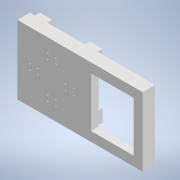
# Autodesk Inventor part: Upper_Half
Saved by Autodesk Inventor 2022 (Build 260153000, 153)
## iProperties
Created: 2023-09-02
Part Number: Upper_Half
Material: Generic
Document SubType Name: Modeling
Designer: Petr Černý
Density: 1 g/cm^3
Appearance: Default
Author: Petr Černý
Autodesk Inventor part; units mm, degrees
ref_plane "YZ Plane" through (0, 0, 0) normal (1, 0, 0) x (0, 1, 0)
ref_plane "XZ Plane" through (0, 0, 0) normal (0, 1, 0) x (-1, 0, 0)
ref_plane "XY Plane" through (0, 0, 0) normal (0, 0, 1) x (1, 0, 0)
sketch "Sketch1" plane through (0, 0, 0) normal (0, 0, 1) x (1, 0, 0)
  line L0 (99.9399, 34.6241) -> (-14.0601, 34.6241)
  line L1 (-14.0601, 34.6241) -> (-14.0601, -20.3759)
  line L2 (-14.0601, -20.3759) -> (99.9399, -20.3759)
  line L3 (99.9399, -20.3759) -> (99.9399, 34.6241)
  point P0 (0, 0)
  dimension "d0" = 114
  dimension "d1" = 55
  constraints: 8 end point, 2 parallel, 1 horizontal, 1 perpendicular
  measures "d0" distance of L1.end L2.end
  measures "d1" distance of L0.end L1.end
extrude "Extrusion1" add sketch "Sketch1" along normal blind 6
shell "Shell1" thickness 2 removed faces 1 at (23.9399, -2.0426, 0)
sketch "Sketch2" plane through (97.9399, 32.6241, 4) normal (0, 0, -1) x (-1, 0, 0)
  line L0 (110, 0) -> (110, -51) projected
  line L1 (0, 0) -> (110, 0) projected
  line L2 (110, 0) -> (110, -51) projected
  line L3 (110, -51) -> (0, -51) projected
  line L4 (0, -51) -> (0, 0) projected
  line L5 (112, 2) -> (112, -53) projected
  line L6 (-2, 2) -> (112, 2) projected
  line L7 (-2, -53) -> (-2, 2) projected
  line L8 (112, -53) -> (-2, -53) projected
  line L9 (110, 0) -> (110, -51) projected
  line L10 (110, 0) -> (100, 0)
  line L11 (100, 0) -> (100, -10)
  line L12 (100, -10) -> (110, -10)
  line L13 (110, -10) -> (110, 0)
  line L14 (110, -51) -> (0, -51) projected
  line L15 (110, -51) -> (100, -51)
  line L16 (100, -51) -> (100, -41)
  line L17 (100, -41) -> (110, -41)
  line L18 (110, -41) -> (110, -51)
  line L19 (0, 0) -> (110, 0) projected
  line L20 (70, 0) -> (60, 0)
  line L21 (60, 0) -> (60, -10)
  line L22 (60, -10) -> (70, -10)
  line L23 (70, -10) -> (70, 0)
  line L24 (70, -51) -> (60, -51)
  line L25 (60, -51) -> (60, -41)
  line L26 (60, -41) -> (70, -41)
  line L27 (70, -41) -> (70, -51)
  point P0 (97.9399, -32.6241)
  point P1 (105, -4.45)
  point P2 (105, -46.55)
  point P3 (65, -4.45)
  point P4 (65, -46.55)
  point P5 (60, 0)
  point P6 (100, 0)
  dimension "d5" = 10
  dimension "d6" = 10
  dimension "d7" = 10
  dimension "d8" = 10
  dimension "d9" = 10
  dimension "d10" = 10
  dimension "d11" = 10
  dimension "d12" = 10
  dimension "d13" = 30
  dimension "d14" = 4.45
  dimension "d15" = 4.45
  dimension "d16" = 42.1
  dimension "d17" = 5
  dimension "d18" = 5
  dimension "d19" = 40
  dimension "d20" = 40
  constraints: 32 end point, 8 parallel, 4 horizontal, 4 perpendicular, 3 point on line
  measures "d5" distance of L12.end L11.end
  measures "d6" distance of L11.end L10.end
  measures "d7" distance of L16.end L17.end
  measures "d8" distance of L15.end L16.end
  measures "d9" distance of L22.end L21.end
  measures "d10" distance of L21.end L20.end
  measures "d11" distance of L25.end L26.end
  measures "d12" distance of L24.end L25.end
  measures "d13" distance between parallel lines of L11 L23
  measures "d14" distance from line of L1 point (105, -4.45)
  measures "d15" distance from line of L3 point (105, -46.55)
  measures "d16" distance of point (105, -46.55) point (105, -4.45)
  measures "d17" distance from line of L0 point (105, -4.45)
  measures "d18" distance from line of L0 point (105, -46.55)
  measures "d19" distance of point (65, -4.45) point (105, -4.45)
  measures "d20" distance of point (65, -46.55) point (105, -46.55)
extrude "Extrusion2" add sketch "Sketch2" along normal blind 14 contours L0 L12 L11 L1 | L0 L3 L16 L17 | L23 L22 L21 L1 | L3 L25 L26 L27
sketch "Sketch3" plane through (0, 0, 0) normal (0, 0, -1) x (-1, 0, 0)
  line L0 (-27.9399, -18.3759) -> (-37.9399, -18.3759) projected
  line L1 (12.0601, -8.3759) -> (12.0601, -18.3759) projected
  line L2 (2.0601, -18.3759) -> (2.0601, -8.3759) projected
  line L3 (-27.9399, -8.3759) -> (-27.9399, -18.3759) projected
  point P0 (0, 0)
  point P1 (7.0601, 28.1741)
  point P2 (7.0601, -13.9259)
  point P3 (-32.9399, -13.9259)
  point P4 (-32.9399, 28.1741)
  point P5 (7.0601, 28.1741)
  point P6 (7.0601, -13.9259)
  point P7 (-32.9399, -13.9259)
  point P8 (-32.9399, 28.1741)
  dimension "d66" = 42.1
  dimension "d67" = 4.45
  dimension "d68" = 40
  dimension "d69" = 5
  dimension "d70" = 30
  constraints: 4 coincident
  measures "d66" distance of point (-32.94, -13.926) point (-32.94, 28.174)
  measures "d67" distance from line of L0 point (-32.94, -13.926)
  measures "d68" distance of point (7.06, -13.926) point (-32.94, -13.926)
  measures "d69" distance from line of L1 point (7.06, -13.926)
  measures "d70" distance between parallel lines of L2 L3
hole "Hole1" at (-7.0601, 28.1741, 0) at (-7.0601, -13.9259, 0) at (32.9399, -13.9259, 0) at (32.9399, 28.1741, 0) direction (0, 0, 1) diameter 2.459 depth 5 tip angle 118 thread size "M3x0.5" class "6H" standard "ISO Metric profile"
sketch "Sketch4" plane through (0, 0, 6) normal (0, 0, 1) x (1, 0, 0)
  line L0 (-14.0601, 34.6241) -> (-14.0601, -20.3759) projected
  line L1 (99.9399, 34.6241) -> (-14.0601, 34.6241) projected
  line L2 (-14.0601, -20.3759) -> (99.9399, -20.3759) projected
  point P0 (0, 0)
  point P1 (-4.0601, 9.3741)
  point P2 (-4.0601, 4.8741)
  point P3 (2.4399, 4.8741)
  point P4 (2.4399, 9.3741)
  point P5 (10.1899, -5.1259)
  point P6 (10.1899, -9.6259)
  point P7 (16.6899, -9.6259)
  point P8 (16.6899, -5.1259)
  point P9 (16.6899, 23.8741)
  point P10 (16.6899, 19.3741)
  point P11 (10.1899, 19.3741)
  point P12 (10.1899, 23.8741)
  point P13 (30.9399, 9.3741)
  point P14 (24.4399, 9.3741)
  point P15 (24.4399, 4.8741)
  point P16 (30.9399, 4.8741)
  dimension "d30" = 4.5
  dimension "d31" = 6.5
  dimension "d32" = 6.5
  dimension "d33" = 10
  dimension "d34" = 25.25
  dimension "d35" = 4.5
  dimension "d36" = 6.5
  dimension "d37" = 6.5
  dimension "d38" = 4.5
  dimension "d39" = 6.5
  dimension "d40" = 6.5
  dimension "d41" = 4.5
  dimension "d42" = 6.5
  dimension "d43" = 6.5
  dimension "d44" = 22
  dimension "d45" = 0
  dimension "d46" = 7.75
  dimension "d47" = 7.75
  dimension "d48" = 10
  dimension "d49" = 10
  measures "d30" distance of point (-4.06, 4.874) point (-4.06, 9.374)
  measures "d31" distance of point (2.44, 9.374) point (-4.06, 9.374)
  measures "d32" distance of point (2.44, 4.874) point (-4.06, 4.874)
  measures "d33" distance from line of L0 point (-4.06, 4.874)
  measures "d34" distance from line of L2 point (-4.06, 4.874)
  measures "d35" distance of point (10.19, -9.626) point (10.19, -5.126)
  measures "d36" distance of point (16.69, -5.126) point (10.19, -5.126)
  measures "d37" distance of point (16.69, -9.626) point (10.19, -9.626)
  measures "d38" distance of point (10.19, 19.374) point (10.19, 23.874)
  measures "d39" distance of point (16.69, 23.874) point (10.19, 23.874)
  measures "d40" distance of point (16.69, 19.374) point (10.19, 19.374)
  measures "d41" distance of point (24.44, 4.874) point (24.44, 9.374)
  measures "d42" distance of point (30.94, 9.374) point (24.44, 9.374)
  measures "d43" distance of point (30.94, 4.874) point (24.44, 4.874)
  measures "d44" distance of point (24.44, 4.874) point (2.44, 4.874)
  measures "d45" vertical distance of point (24.44, 4.874) point (2.44, 4.874)
  measures "d46" horizontal distance of point (10.19, -9.626) point (2.44, 4.874)
  measures "d47" horizontal distance of point (10.19, 19.374) point (2.44, 9.374)
  measures "d48" vertical distance of point (2.44, 9.374) point (10.19, 19.374)
  measures "d49" vertical distance of point (10.19, -5.126) point (2.44, 4.874)
hole "Hole2" at (-4.0601, 9.3741, 6) at (-4.0601, 4.8741, 6) at (2.4399, 4.8741, 6) at (2.4399, 9.3741, 6) at (16.6899, -5.1259, 6) at (16.6899, -9.6259, 6) at (10.1899, -9.6259, 6) at (10.1899, -5.1259, 6) at (16.6899, 23.8741, 6) at (10.1899, 23.8741, 6) at (10.1899, 19.3741, 6) at (16.6899, 19.3741, 6) at (30.9399, 4.8741, 6) at (24.4399, 4.8741, 6) at (24.4399, 9.3741, 6) at (30.9399, 9.3741, 6) direction (0, 0, -1) diameter 1 end through all
sketch "Sketch5" plane through (97.9399, -18.3759, 4) normal (0, 0, -1) x (-1, 0, 0)
  line L0 (0, 0) -> (0, 51) projected
  line L1 (0, 0) -> (46.7, 0)
  line L2 (46.7, 0) -> (46.7, 51)
  line L3 (46.7, 51) -> (0, 51)
  line L4 (0, 51) -> (0, 0)
  point P0 (97.9399, 18.3759)
  point P1 (0, 51)
  dimension "d57" = 46.7
  constraints: 8 end point, 2 parallel, 1 horizontal, 1 perpendicular
  measures "d57" distance of L3.end L2.end
extrude "Extrusion3" add sketch "Sketch5" along normal blind 2
sketch "Sketch6" plane through (97.9399, -18.3759, 2) normal (0, 0, -1) x (-1, 0, 0)
  line L0 (5.2, 5.55) -> (39.2, 5.55)
  line L1 (39.2, 5.55) -> (39.2, 45.45)
  line L2 (39.2, 45.45) -> (5.2, 45.45)
  line L3 (5.2, 45.45) -> (5.2, 5.55)
  line L4 (0, 0) -> (0, 51) projected
  line L5 (60, 0) -> (0, 0) projected
  line L6 (0, 51) -> (60, 51) projected
  point P0 (97.9399, 18.3759)
  dimension "d60" = 34
  dimension "d61" = 39.9
  dimension "d62" = 5.55
  dimension "d63" = 5.2
  constraints: 8 end point, 2 parallel, 1 horizontal, 1 perpendicular
  measures "d60" distance of L2.end L1.end
  measures "d61" distance of L1.end L0.end
  measures "d62" distance between parallel lines of L5 L0
  measures "d63" distance between parallel lines of L3 L4
extrude "Extrusion4" cut sketch "Sketch6" against normal through all
body "Solid1"
